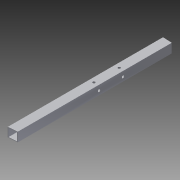
# Autodesk Inventor part: Square Motor Mount
Saved by Autodesk Inventor 2013 (Build 170138000, 138)
## iProperties
Created: 2013-01-21
Part Number: Square Motor Mount
Material: Aluminum 6061
Document SubType Name: Modeling
Designer: actoennies
Density: 2.71 g/cm^3
Mass: 178.467 g
Surface Area: 835.389 cm^2
Volume: 65.8549 cm^3
Author: actoennies
Autodesk Inventor part; units mm, degrees
ref_plane "YZ Plane" through (0, 0, 0) normal (1, 0, 0) x (0, 1, 0)
ref_plane "XZ Plane" through (0, 0, 0) normal (0, 1, 0) x (-1, 0, 0)
ref_plane "XY Plane" through (0, 0, 0) normal (0, 0, 1) x (1, 0, 0)
sketch "Sketch1" plane through (0, 0, 0) normal (0, 0, 1) x (1, 0, 0)
  line L0 (0, 0) -> (-25.4, 0)
  line L1 (-25.4, 0) -> (-25.4, 25.4)
  line L2 (-25.4, 25.4) -> (0, 25.4)
  line L3 (0, 25.4) -> (0, 0)
  line L4 (-1.5875, 23.8125) -> (-23.8125, 23.8125)
  line L5 (-23.8125, 23.8125) -> (-23.8125, 1.5875)
  line L6 (-23.8125, 1.5875) -> (-1.5875, 1.5875)
  line L7 (-1.5875, 1.5875) -> (-1.5875, 23.8125)
  dimension "d0" = 25.4
  dimension "d2" = 25.4
  dimension "d3" = 1.5875
  constraints: 16 end point, 4 parallel, 2 perpendicular, 1 horizontal, 3 other
  measures "d0" distance of L1.end L2.end
  measures "d2" distance of L2.end L0.start
  measures "d3" distance between parallel lines of L2 L4
extrude "Extrusion1" add sketch "Sketch1" along normal blind 508
sketch "Sketch2" plane through (-25.4, 25.4, 0) normal (0, 1, 0) x (1, 0, 0)
  line L0 (0, 0) -> (25.4, 0) projected
  line L1 (0, 0) -> (0, -508) projected
  line L2 (25.4, -508) -> (0, -508) projected
  line L3 (25.4, 0) -> (25.4, -508) projected
  line L4 (0, -63.5) -> (25.4, -63.5) construction
  line L5 (0, -63.5) -> (25.4, -63.5)
  point P0 (25.4, -54.61)
  point P1 (0, -56.388)
  point P2 (25.4, -60.1453)
  dimension "d12" = 3.3547
  dimension "d13" = 444.5
  constraints: 5 point on line, 4 end point, 1 collinear, 1 perpendicular
  measures "d12" distance of L4.end point (25.4, -60.145)
  measures "d13" distance from line of L2 L4.start
extrude "Extrusion2" cut sketch "Sketch2" against normal blind 508 contours L0 L3 L5 L1
sketch "Sketch3" plane through (-25.4, 0, 508) normal (0, -1, 0) x (1, 0, 0)
  circle A0 centre (12.7, -235.8157) radius 3.3782
  circle A1 centre (12.7, -305.6657) radius 3.3782
  point P0 (25.4, -508)
  constraints: 2 centre point, 4 other
extrude "Extrusion3" cut sketch "Sketch3" against normal blind 25.4
sketch "Sketch4" plane through (0, 0, 508) normal (1, 0, 0) x (0, 0, -1)
  circle A0 centre (237.4032, 11.3284) radius 3.3782
  circle A1 centre (303.4032, 11.3284) radius 3.3782
  point P0 (508, 0)
  constraints: 2 centre point, 4 other
extrude "Extrusion4" cut sketch "Sketch4" against normal blind 25.4
sketch "Sketch5" plane through (-25.4, 25.4, 508) normal (0, 1, 0) x (1, 0, 0)
  line L0 (25.4, 444.5) -> (0, 444.5) projected
  line L1 (0, 444.5) -> (0, 0) projected
  line L2 (25.4, 444.5) -> (25.4, 0) projected
  line L3 (25.4, 437.9919) -> (0, 439.0728)
  line L4 (0, 439.0728) -> (0, 444.5)
  line L5 (0, 444.5) -> (25.4, 444.5)
  line L6 (25.4, 444.5) -> (25.4, 437.9919)
  point P0 (25.4, 508)
  constraints: 8 end point, 2 point on line, 1 collinear, 1 perpendicular, 3 other
extrude "Extrusion5" cut sketch "Sketch5" against normal blind 25.4
sketch "Sketch6" plane through (-25.4, 25.4, 508) normal (0, 1, 0) x (1, 0, 0)
  line L0 (0, 439.0728) -> (0, 0) projected
  line L1 (25.4, 0) -> (0, 0) projected
  line L2 (25.4, 437.9919) -> (25.4, 0) projected
  line L3 (469.9, 50.8918) -> (-127, 0.0918)
  line L4 (469.9, 50.8918) -> (-127, 0.0918)
  line L5 (25.4, 13.062) -> (0, 10.9003)
  point P0 (25.4, 508)
  constraints: 6 end point, 4 point on line, 4 other
extrude "Extrusion6" cut sketch "Sketch6" against normal blind 25.4
body "Solid1"
